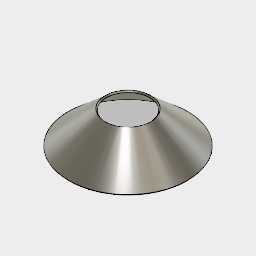
assembled (Autodesk Fusion 360 archive; units mm, degrees)
design "top_roof"
Autodesk Fusion 360 part; units mm, degrees
sketch "スケッチ1" plane through (0, 0, 0) normal (0, 0, 1) x (1, 0, 0)
  line L0 (0, 0) -> (0, 35)
  line L1 (0, 35) -> (30, 35)
  line L2 (0, 0) -> (70, 0)
  line L3 (30, 35) -> (70, 0)
  line L4 (70, 0) -> (132.0268, -54.2735)
  line L5 (0, 0) -> (0, -10)
  line L6 (0, -10) -> (81.4286, -10)
  line L7 (30, 35) -> (81.4286, -10)
  line L8 (81.4286, -10) -> (83.0748, -8.1186)
  line L9 (83.0748, -8.1186) -> (31.6463, 36.8814)
  line L10 (31.6463, 36.8814) -> (30, 35)
  dimension "d1" = 35
  dimension "d2" = 30
  dimension "d3" = 70
  dimension "d4" = 10
  dimension "d5" = 2.5
  measures "d1" distance of L0.start L0.end
  measures "d2" distance of L0.end L1.end
  measures "d3" distance of L0.start L2.end
  measures "d4" distance of L0.start L5.end
  measures "d5" distance of L1.end L9.end
revolve "回転1" add sketch "スケッチ1" angle 360 about axis through (0, 0, 0) along (0, 1, 0) contours L3 L4 L7 L8 L9 L10

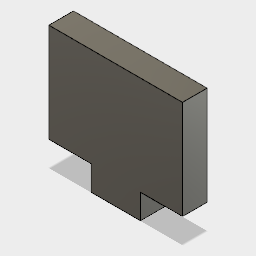
design "servo_guide3"
Autodesk Fusion 360 part; units mm, degrees
sketch "スケッチ1" plane through (0, 0, 0) normal (0, 0, 1) x (1, 0, 0)
  line L0 (173.9056, -200.0792) -> (173.9056, -202.5793)
  line L1 (183.1559, -190.0791) -> (169.639, -190.0791)
  line L2 (169.639, -200.0792) -> (173.9056, -200.0792)
  line L3 (178.9056, -202.5793) -> (178.9056, -200.0792)
  line L4 (178.9056, -200.0792) -> (183.1559, -200.0792)
  line L5 (169.639, -190.0791) -> (169.639, -200.0792)
  line L6 (173.9056, -202.5793) -> (178.9056, -202.5793)
  line L7 (183.1559, -200.0792) -> (183.1559, -190.0791)
extrude "押し出し1" add sketch "スケッチ1" along normal blind 2.5

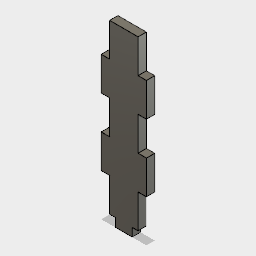
design "servo_guide2"
Autodesk Fusion 360 part; units mm, degrees
sketch "スケッチ1" plane through (0, 0, 0) normal (0, 0, 1) x (1, 0, 0)
  line L0 (35.16, -63.4696) -> (35.16, -53.4695)
  line L1 (35.16, -53.4695) -> (32.66, -53.4695)
  line L2 (32.66, -53.4695) -> (32.66, -43.4694)
  line L3 (32.66, -43.4694) -> (35.16, -43.4694)
  line L4 (35.16, -43.4694) -> (35.16, -33.4693)
  line L5 (35.16, -33.4693) -> (32.66, -33.4693)
  line L6 (32.66, -33.4693) -> (32.66, -23.4692)
  line L7 (32.66, -23.4692) -> (35.16, -23.4692)
  line L8 (35.16, -23.4692) -> (35.16, -13.4691)
  line L9 (35.16, -13.4691) -> (43.6602, -13.4691)
  line L10 (43.6602, -13.4691) -> (43.6602, -23.4692)
  line L11 (43.6602, -23.4692) -> (46.1602, -23.4692)
  line L12 (46.1602, -23.4692) -> (46.1602, -33.4693)
  line L13 (46.1602, -33.4693) -> (43.6602, -33.4693)
  line L14 (43.6602, -33.4693) -> (43.6602, -43.4694)
  line L15 (43.6602, -43.4694) -> (46.1602, -43.4694)
  line L16 (46.1602, -43.4694) -> (46.1602, -53.4695)
  line L17 (46.1602, -53.4695) -> (43.6602, -53.4695)
  spline S0 degree 3 poles (43.6602, -53.4695) (43.6602, -53.4695) (43.6602, -63.4696) (43.6601, -63.4696) knots 18 18 18 18 19 19 19 19
  line L18 (43.6601, -63.4696) -> (41.9101, -63.4696)
  line L19 (41.9101, -63.4696) -> (41.9101, -65.9695)
  line L20 (41.9101, -65.9695) -> (36.9101, -65.9695)
  line L21 (36.9101, -65.9695) -> (36.9101, -63.4696)
  line L22 (36.9101, -63.4696) -> (35.16, -63.4696)
extrude "押し出し1" add sketch "スケッチ1" along normal blind 2.5

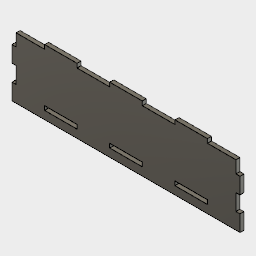
design "base_frontside"
Autodesk Fusion 360 part; units mm, degrees
sketch "スケッチ1" plane through (0, 0, 0) normal (0, 0, 1) x (1, 0, 0)
  line L0 (227.26, -118.9783) -> (227.26, -121.4783)
  line L1 (127.2604, -118.9783) -> (147.2604, -118.9783)
  line L2 (227.26, -121.4783) -> (207.2598, -121.4783)
  line L3 (147.2604, -118.9783) -> (147.2604, -121.4783)
  line L4 (207.2598, -121.4783) -> (207.2598, -118.9783)
  line L5 (187.2604, -121.4783) -> (167.2602, -121.4783)
  line L6 (207.2598, -118.9783) -> (227.26, -118.9783)
  line L7 (187.2604, -118.9783) -> (187.2604, -121.4783)
  line L8 (167.2602, -121.4783) -> (167.2602, -118.9783)
  line L9 (167.2602, -118.9783) -> (187.2604, -118.9783)
  line L10 (244.7608, -88.9781) -> (227.2604, -88.9781)
  line L11 (227.2604, -88.9781) -> (227.2604, -86.478)
  line L12 (227.2604, -86.478) -> (207.2605, -86.478)
  line L13 (207.2605, -86.478) -> (207.2605, -88.9781)
  line L14 (207.2605, -88.9781) -> (187.2604, -88.9781)
  line L15 (187.2604, -88.9781) -> (187.2604, -86.478)
  line L16 (187.2604, -86.478) -> (167.2604, -86.478)
  line L17 (167.2604, -86.478) -> (167.2604, -88.9781)
  line L18 (167.2604, -88.9781) -> (147.2604, -88.9781)
  line L19 (147.2604, -88.9781) -> (147.2604, -86.478)
  line L20 (147.2604, -86.478) -> (127.2604, -86.478)
  line L21 (127.2604, -86.478) -> (127.2604, -88.9781)
  line L22 (127.2604, -88.9781) -> (109.7603, -88.9781)
  line L23 (109.7603, -88.9781) -> (109.7603, -96.4781)
  line L24 (109.7603, -96.4781) -> (107.2604, -96.4781)
  line L25 (107.2604, -96.4781) -> (107.2604, -106.4782)
  line L26 (107.2604, -106.4782) -> (109.7603, -106.4782)
  line L27 (109.7603, -106.4782) -> (109.7603, -116.4782)
  line L28 (109.7603, -116.4782) -> (107.2604, -116.4782)
  line L29 (107.2604, -116.4782) -> (107.2604, -126.4783)
  line L30 (107.2604, -126.4783) -> (109.7603, -126.4783)
  line L31 (109.7603, -126.4783) -> (244.7608, -126.4783)
  line L32 (244.7608, -126.4783) -> (247.2605, -126.4783)
  line L33 (247.2605, -126.4783) -> (247.2605, -116.4782)
  line L34 (247.2605, -116.4782) -> (244.7608, -116.4782)
  line L35 (244.7608, -116.4782) -> (244.7608, -106.4782)
  line L36 (244.7608, -106.4782) -> (247.2605, -106.4782)
  line L37 (247.2605, -106.4782) -> (247.2605, -96.4781)
  line L38 (247.2605, -96.4781) -> (244.7608, -96.4781)
  line L39 (244.7608, -96.4781) -> (244.7608, -88.9781)
  line L40 (147.2604, -121.4783) -> (127.2604, -121.4783)
  line L41 (127.2604, -121.4783) -> (127.2604, -118.9783)
extrude "押し出し1" add sketch "スケッチ1" along normal blind 2.5

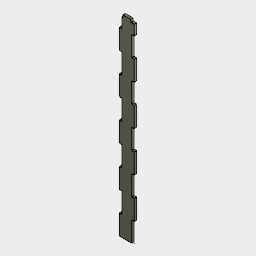
design "pillar"
Autodesk Fusion 360 part; units mm, degrees
sketch "スケッチ1" plane through (0, 0, 0) normal (0, 0, 1) x (1, 0, 0)
  line L0 (20.0472, -16.9044) -> (20.0472, -26.9043)
  line L1 (20.0472, -26.9043) -> (17.5473, -26.9043)
  line L2 (17.5473, -26.9043) -> (17.5473, -46.9043)
  line L3 (17.5473, -46.9043) -> (20.0472, -46.9043)
  line L4 (20.0472, -46.9043) -> (20.0472, -66.9043)
  line L5 (20.0472, -66.9043) -> (17.5473, -66.9043)
  line L6 (17.5473, -66.9043) -> (17.5473, -86.9043)
  line L7 (17.5473, -86.9043) -> (20.0472, -86.9043)
  line L8 (20.0472, -86.9043) -> (20.0472, -106.9043)
  line L9 (20.0472, -106.9043) -> (17.5473, -106.9043)
  line L10 (17.5473, -106.9043) -> (17.5473, -126.9043)
  line L11 (17.5473, -126.9043) -> (20.0472, -126.9043)
  line L12 (20.0472, -126.9043) -> (20.0472, -146.9043)
  line L13 (20.0472, -146.9043) -> (17.5473, -146.9043)
  line L14 (17.5473, -146.9043) -> (17.5473, -166.9043)
  line L15 (17.5473, -166.9043) -> (20.0472, -166.9043)
  line L16 (20.0472, -166.9043) -> (20.0472, -186.9045)
  line L17 (20.0472, -186.9045) -> (17.5473, -186.9045)
  line L18 (17.5473, -186.9045) -> (17.5473, -206.9043)
  spline S0 degree 3 poles (17.5473, -206.9043) (17.5473, -206.9046) (30.0472, -206.9046) (30.0473, -206.9046) knots 19 19 19 19 20 20 20 20
  line L19 (30.0473, -206.9046) -> (30.0473, -186.9045)
  line L20 (30.0473, -186.9045) -> (32.5472, -186.9045)
  line L21 (32.5472, -186.9045) -> (32.5472, -166.9043)
  line L22 (32.5472, -166.9043) -> (30.0473, -166.9043)
  line L23 (30.0473, -166.9043) -> (30.0473, -146.9043)
  line L24 (30.0473, -146.9043) -> (32.5472, -146.9043)
  line L25 (32.5472, -146.9043) -> (32.5472, -126.9043)
  line L26 (32.5472, -126.9043) -> (30.0473, -126.9043)
  line L27 (30.0473, -126.9043) -> (30.0473, -106.9043)
  line L28 (30.0473, -106.9043) -> (32.5472, -106.9043)
  line L29 (32.5472, -106.9043) -> (32.5472, -86.9043)
  line L30 (32.5472, -86.9043) -> (30.0473, -86.9043)
  line L31 (30.0473, -86.9043) -> (30.0473, -66.9043)
  line L32 (30.0473, -66.9043) -> (32.5472, -66.9043)
  line L33 (32.5472, -66.9043) -> (32.5472, -46.9043)
  line L34 (32.5472, -46.9043) -> (30.0473, -46.9043)
  line L35 (30.0473, -46.9043) -> (30.0473, -26.9043)
  line L36 (30.0473, -26.9043) -> (32.5472, -26.9043)
  line L37 (32.5472, -26.9043) -> (32.5472, -16.9044)
  line L38 (32.5472, -16.9044) -> (29.0473, -16.9044)
  line L39 (29.0473, -16.9044) -> (29.0473, -14.4045)
  line L40 (29.0473, -14.4045) -> (21.0473, -14.4045)
  line L41 (21.0473, -14.4045) -> (21.0473, -16.9044)
  line L42 (21.0473, -16.9044) -> (20.0472, -16.9044)
extrude "押し出し1" add sketch "スケッチ1" along normal blind 2.5

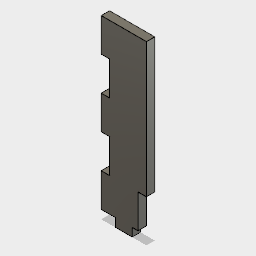
design "servo_guide1"
Autodesk Fusion 360 part; units mm, degrees
sketch "スケッチ1" plane through (0, 0, 0) normal (0, 0, 1) x (1, 0, 0)
  line L0 (19.2851, -21.7594) -> (19.2851, -31.7595)
  line L1 (19.2851, -31.7595) -> (16.7852, -31.7595)
  line L2 (16.7852, -21.7594) -> (19.2851, -21.7594)
  line L3 (16.7852, -41.7596) -> (19.2851, -41.7596)
  line L4 (16.7852, -31.7595) -> (16.7852, -41.7596)
  line L5 (16.7852, -11.7593) -> (16.7852, -21.7594)
  line L6 (21.0353, -61.7598) -> (21.0353, -64.2597)
  line L7 (19.2851, -41.7596) -> (19.2851, -51.7597)
  line L8 (30.2852, -11.7593) -> (16.7852, -11.7593)
  line L9 (21.0353, -64.2597) -> (26.0353, -64.2597)
  line L10 (27.7852, -51.7597) -> (30.2852, -51.7597)
  line L11 (26.0353, -61.7598) -> (27.7852, -61.7598)
  line L12 (16.7852, -51.7597) -> (16.7852, -61.7598)
  line L13 (16.7852, -61.7598) -> (21.0353, -61.7598)
  line L14 (19.2851, -51.7597) -> (16.7852, -51.7597)
  line L15 (26.0353, -64.2597) -> (26.0353, -61.7598)
  line L16 (27.7852, -61.7598) -> (27.7852, -51.7597)
  line L17 (30.2852, -51.7597) -> (30.2852, -11.7593)
extrude "押し出し1" add sketch "スケッチ1" along normal blind 2.5
